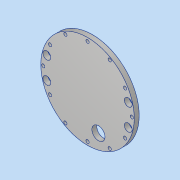
# Autodesk Inventor part: AluminumSealingDiscMidshipsRear
Saved by Autodesk Inventor 2017 (Build 210142000, 142)
## iProperties
Created: 2016-10-25
Part Number: AluminumSealingDiscMidshipsRear
Material: Aluminum 6061
Document SubType Name: Modeling
Designer: techn
Density: 2.7 g/cm^3
Appearance: Aluminum - Flat
Mass: 77.3802 g
Surface Area: 146.044 cm^2
Volume: 28.6593 cm^3
Author: techn
Autodesk Inventor part; units mm, degrees
ref_plane "YZ Plane" through (0, 0, 0) normal (1, 0, 0) x (0, 1, 0)
ref_plane "XZ Plane" through (0, 0, 0) normal (0, 1, 0) x (-1, 0, 0)
ref_plane "XY Plane" through (0, 0, 0) normal (0, 0, 1) x (1, 0, 0)
sketch "Sketch1" plane through (0, 0, 0) normal (0, 0, 1) x (1, 0, 0)
  circle A0 centre (0, 0) radius 45.212
  dimension "d0" = 90.424
  constraints: 1 centre point, 1 coincident
  measures "d0" diameter of A0
extrude "Extrusion1" add sketch "Sketch1" along normal blind 4.7625
sketch "Sketch6" plane through (0, 0, 4.7625) normal (0, 0, 1) x (1, 0, 0)
  circle A0 centre (10.541, -29.7561) radius 6.35
  point P0 (0, 0)
  dimension "d27" = 12.7
  dimension "d28" = 29.7561
  dimension "d29" = 10.541
  constraints: 1 centre point
  measures "d27" diameter of A0
  measures "d28" vertical distance of A0.centre point (0, 0)
  measures "d29" horizontal distance of A0.centre point (0, 0)
extrude "Extrusion6" cut sketch "Sketch6" against normal blind 25.4
sketch "Sketch7" plane through (0, 0, 4.7625) normal (0, 0, 1) x (1, 0, 0)
  line L0 (0, 0) -> (21.4313, 37.12)
  line L1 (0, 0) -> (42.8625, 0) construction
  circle A0 centre (21.4313, 37.12) radius 1.5875
  circle A1 centre (-21.4312, 37.12) radius 1.5875
  circle A2 centre (-42.8625, 0) radius 1.5875
  circle A3 centre (-21.4313, -37.12) radius 1.5875
  circle A4 centre (21.4312, -37.12) radius 1.5875
  circle A5 centre (42.8625, 0) radius 1.5875
  dimension "d32" = 42.8625
  dimension "d33" = 60
  dimension "d34" = 3.175
  dimension "d37" = 360
  constraints: 6 centre point, 4 end point, 1 coincident, 1 equal length, 1 horizontal, 13 other
  measures "d32" distance of L0.start L0.end
  measures "d33" angle of L1 L0
  measures "d34" diameter of A0
extrude "Extrusion7" cut sketch "Sketch7" against normal blind 25.4
sketch "Sketch8" plane through (0, 0, 4.7625) normal (0, 0, 1) x (1, 0, 0)
  line L0 (0, 0) -> (0, 41.91)
  circle A0 centre (0, 41.91) radius 1.5875
  circle A1 centre (-36.2951, 20.955) radius 1.5875
  circle A2 centre (-36.2951, -20.955) radius 1.5875
  circle A3 centre (0, -41.91) radius 1.5875
  circle A4 centre (36.2951, -20.955) radius 1.5875
  circle A5 centre (36.2951, 20.955) radius 1.5875
  dimension "d41" = 41.91
  dimension "d42" = 3.175
  dimension "d45" = 360
  constraints: 6 centre point, 2 end point, 1 coincident, 1 vertical, 13 other
  measures "d41" distance of L0.start L0.end
  measures "d42" diameter of A0
extrude "Extrusion8" cut sketch "Sketch8" against normal blind 25.4
sketch "Sketch10" plane through (0, 0, 4.7625) normal (0, 0, 1) x (1, 0, 0)
  line L0 (0, 0) -> (39.3779, 10.5513)
  line L1 (0, 0) -> (40.767, 0) construction
  circle A0 centre (39.3779, 10.5513) radius 3.81
  line L2 (0, 0) -> (0, 16.2318)
  circle A1 centre (39.3779, -10.5513) radius 3.81
  circle A2 centre (-39.3779, 10.5513) radius 3.81
  circle A3 centre (-39.3779, -10.5513) radius 3.81
  dimension "d49" = 40.767
  dimension "d50" = 15
  dimension "d51" = 7.62
  constraints: 6 end point, 4 centre point, 3 symmetric about line, 1 coincident, 1 equal length, 1 horizontal, 1 vertical, 3 other
  measures "d49" distance of L0.start L0.end
  measures "d50" angle of L1 L0
  measures "d51" diameter of A0
extrude "Extrusion9" cut sketch "Sketch10" against normal blind 25.4
body "Solid1"
